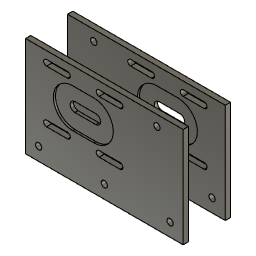
Nema 24 rear mount plate v10 (Autodesk Fusion 360 design; units mm, degrees)
Autodesk Fusion 360 part; units mm, degrees
sketch "Sketch1" plane through (0, 0, 0) normal (0, 1, 0) x (1, 0, 0)
  line L0 (0, 0) -> (150, 0)
  line L1 (150, 0) -> (150, -95)
  line L2 (150, -95) -> (0, -95)
  line L3 (0, -95) -> (0, 0)
  circle A0 centre (125, -85) radius 3
  circle A1 centre (137.5, -12.5) radius 3
  circle A2 centre (75, -12.5) radius 3
  circle A3 centre (12.5, -12.5) radius 3
  circle A4 centre (20, -85) radius 2.75
  line L4 (40, -82.25) -> (20, -82.25)
  line L5 (20.0062, -87.75) -> (40, -87.75)
  circle A5 centre (40, -85) radius 2.75
  circle A6 centre (70, -85) radius 2.75
  line L6 (70, -82.25) -> (90, -82.25)
  line L7 (90, -87.75) -> (70, -87.75)
  circle A7 centre (90, -85) radius 2.75
  circle A8 centre (20, -35) radius 2.75
  line L8 (40, -32.25) -> (20, -32.25)
  line L9 (20, -37.75) -> (40, -37.75)
  circle A9 centre (40, -35) radius 2.75
  circle A10 centre (70, -35) radius 2.75
  line L10 (90, -32.25) -> (70, -32.25)
  line L11 (70, -37.75) -> (90, -37.75)
  circle A11 centre (90, -35) radius 2.75
  line L12 (45, -55.5) -> (65, -55.5)
  line L13 (65, -64.5) -> (45, -64.5)
  circle A12 centre (45, -60) radius 4.5
  circle A13 centre (65, -60) radius 4.5
  circle A14 centre (45, -60) radius 18.5
  line L14 (65.0006, -41.5) -> (45, -41.5)
  circle A15 centre (65, -60) radius 18.5
  line L15 (65.0006, -78.5) -> (45, -78.5)
  dimension "d1" = 150
  dimension "d2" = 95
  dimension "d33" = 6
  dimension "d34" = 6
  dimension "d35" = 6
  dimension "d36" = 6
  dimension "d37" = 5.5
  dimension "d38" = 5.5
  dimension "d39" = 5.5
  dimension "d40" = 5.5
  dimension "d41" = 5.5
  dimension "d42" = 5.5
  dimension "d43" = 5.5
  dimension "d44" = 5.5
  dimension "d45" = 9
  dimension "d46" = 9
  dimension "d49" = 37
  dimension "d50" = 37
  constraint horizontal L0
  constraint vertical L1
  constraint horizontal L2
  constraint vertical L3
  constraint coincident L0.start L3.end
  constraint coincident L5.start A4
  constraint coincident L5.end A5
  constraint tangent L5 A5
  constraint coincident L4.start A5
  constraint coincident L4.end A4
  constraint tangent A4 L4
  constraint horizontal L4
  constraint coincident L7.start A7
  constraint coincident L7.end A6
  constraint tangent A6 L7
  constraint coincident L6.start A6
  constraint coincident L6.end A7
  constraint tangent L6 A7
  constraint parallel L6 L7
  constraint coincident L8.end A8
  constraint tangent A8 L8
  constraint coincident L9.start A8
  constraint coincident L9.end A9
  constraint tangent L9 A9
  constraint parallel L8 L9
  constraint coincident L11.start A10
  constraint coincident L11.end A11
  constraint tangent L11 A11
  constraint coincident L10.start A11
  constraint coincident L10.end A10
  constraint tangent A10 L10
  constraint coincident L12.start A12
  constraint coincident L12.end A13
  constraint tangent L12 A13
  constraint horizontal L12
  constraint coincident L13.start A13
  constraint coincident L13.end A12
  constraint tangent L13 A12
  constraint parallel L12 L13
  constraint coincident L15.start A15
  constraint coincident L15.end A14
  constraint tangent A14 L15
  constraint coincident L14.start A15
  constraint coincident L14.end A14
  constraint tangent A14 L14
  measures "d1" distance of L0.start L0.end
  measures "d2" distance of L0.start L2.end
  measures "d33" diameter of A0
  measures "d34" diameter of A1
  measures "d35" diameter of A2
  measures "d36" diameter of A3
  measures "d37" diameter of A5
  measures "d38" diameter of A4
  measures "d39" diameter of A7
  measures "d40" diameter of A6
  measures "d41" diameter of A9
  measures "d42" diameter of A8
  measures "d43" diameter of A11
  measures "d44" diameter of A10
  measures "d45" diameter of A13
  measures "d46" diameter of A12
  measures "d49" diameter of A15
  measures "d50" diameter of A14
sketch "Sketch2" plane through (0, 0, 0) normal (0, 1, 0) x (1, 0, 0)
  line L0 (0, 0) -> (150, 0)
  line L1 (150, 0) -> (150, -25)
  line L2 (150, -25) -> (0, -25)
  line L3 (0, -25) -> (0, 0)
  circle A0 centre (137.5, -12.5) radius 3
  circle A1 centre (12.5, -12.5) radius 3
  circle A2 centre (75, -12.5) radius 3
  dimension "d3" = 150
  dimension "d4" = 25
  dimension "d19" = 6
  dimension "d20" = 6
  dimension "d21" = 6
  constraint horizontal L0
  constraint vertical L1
  constraint horizontal L2
  constraint vertical L3
  constraint coincident L0.start L3.end
  measures "d3" distance of L0.start L0.end
  measures "d4" distance of L0.start L2.end
  measures "d19" diameter of A0
  measures "d20" diameter of A1
  measures "d21" diameter of A2
sketch "Sketch3" plane through (0, 0, 0) normal (0, 1, 0) x (1, 0, 0)
  line L0 (150, -25) -> (100, -25)
  line L1 (100, -25) -> (100, -75)
  line L2 (100, -75) -> (150, -75)
  line L3 (150, -75) -> (150, -25)
  line L4 (100, -75) -> (150, -75)
  line L5 (150, -75) -> (150, -110)
  line L6 (150, -110) -> (100, -110)
  line L7 (100, -110) -> (100, -75)
  circle A0 centre (125, -85) radius 3
  point P0 (150, -25)
  dimension "d5" = 50
  dimension "d6" = 50
  dimension "d7" = 50
  dimension "d8" = 35
  dimension "d22" = 6
  constraint horizontal L0
  constraint vertical L1
  constraint horizontal L2
  constraint vertical L3
  constraint coincident P0 L0.start
  constraint horizontal L4
  constraint vertical L5
  constraint horizontal L6
  constraint vertical L7
  measures "d5" distance of P0 L0.end
  measures "d6" distance of P0 L2.end
  measures "d7" distance of L1.end L2.end
  measures "d8" distance of L1.end L6.end
  measures "d22" diameter of A0
sketch "Sketch4" plane through (0, 0, 0) normal (0, 1, 0) x (1, 0, 0)
  line L0 (95, -30) -> (15, -30)
  line L1 (15, -30) -> (15, -90)
  line L2 (15, -90) -> (95, -90)
  line L3 (95, -90) -> (95, -30)
  circle A0 centre (65, -60) radius 4.5
  circle A1 centre (65, -60) radius 18.5
  circle A2 centre (40, -85) radius 2.75
  circle A3 centre (90, -85) radius 2.75
  circle A4 centre (40, -35) radius 2.75
  circle A5 centre (90, -35) radius 2.75
  circle A6 centre (20, -35) radius 2.75
  circle A7 centre (20, -85) radius 2.75
  circle A8 centre (70, -85) radius 2.75
  circle A9 centre (70, -35) radius 2.75
  line L4 (20.0062, -87.75) -> (40, -87.75)
  line L5 (40, -82.25) -> (20, -82.25)
  line L6 (90, -87.75) -> (70, -87.75)
  line L7 (70, -82.25) -> (90, -82.25)
  line L8 (70, -37.75) -> (90, -37.75)
  line L9 (90, -32.25) -> (70, -32.25)
  line L10 (40, -32.25) -> (20, -32.25)
  line L11 (20, -37.75) -> (40, -37.75)
  circle A10 centre (45, -60) radius 4.5
  circle A11 centre (45, -60) radius 18.5
  line L12 (65.0006, -78.5) -> (45, -78.5)
  line L13 (65.0006, -41.5) -> (45, -41.5)
  line L14 (45, -55.5) -> (65, -55.5)
  line L15 (65, -64.5) -> (45, -64.5)
  dimension "d9" = 80
  dimension "d10" = 60
  dimension "d11" = 9
  dimension "d12" = 37
  dimension "d13" = 5.5
  dimension "d14" = 5.5
  dimension "d15" = 5.5
  dimension "d16" = 5.5
  dimension "d23" = 5.5
  dimension "d24" = 5.5
  dimension "d25" = 5.5
  dimension "d26" = 5.5
  dimension "d27" = 9
  dimension "d28" = 37
  constraint horizontal L0
  constraint vertical L1
  constraint horizontal L2
  constraint vertical L3
  constraint concentric A0 A1
  constraint coincident A7 L4.start
  constraint coincident A2 L4.end
  constraint tangent A2 L4
  constraint coincident A2 L5.start
  constraint coincident A7 L5.end
  constraint tangent A7 L5
  constraint horizontal L5
  constraint coincident A3 L6.start
  constraint coincident A8 L6.end
  constraint tangent A8 L6
  constraint perpendicular L3 L6
  constraint coincident A8 L7.start
  constraint coincident A3 L7.end
  constraint tangent A3 L7
  constraint parallel L6 L7
  constraint coincident A9 L8.start
  constraint coincident A5 L8.end
  constraint tangent A5 L8
  constraint parallel L2 L8
  constraint coincident A5 L9.start
  constraint coincident A9 L9.end
  constraint tangent A9 L9
  constraint parallel L2 L9
  constraint coincident A6 L10.end
  constraint tangent A6 L10
  constraint parallel L0 L10
  constraint coincident A6 L11.start
  constraint coincident A4 L11.end
  constraint tangent A4 L11
  constraint parallel L10 L11
  constraint coincident A1 L12.start
  constraint coincident A11 L12.end
  constraint tangent A11 L12
  constraint coincident A1 L13.start
  constraint coincident A11 L13.end
  constraint tangent A11 L13
  constraint coincident A10 L14.start
  constraint coincident A0 L14.end
  constraint tangent A0 L14
  constraint horizontal L14
  constraint coincident A0 L15.start
  constraint coincident A10 L15.end
  constraint tangent A10 L15
  constraint parallel L14 L15
  measures "d9" distance of L0.start L0.end
  measures "d10" distance of L0.start L2.end
  measures "d11" diameter of A0
  measures "d12" diameter of A1
  measures "d13" diameter of A2
  measures "d14" diameter of A3
  measures "d15" diameter of A4
  measures "d16" diameter of A5
  measures "d23" diameter of A6
  measures "d24" diameter of A7
  measures "d25" diameter of A8
  measures "d26" diameter of A9
  measures "d27" diameter of A10
  measures "d28" diameter of A11
extrude "Extrude4" add sketch "Sketch1" along normal blind 5 contours L0 L1 L2 L3 | L12 L13 A12 A14 A15 | L12 A14 A15 | L12 L13 A13 A14 A15 | A14 L14 A15 | L13 A14 A15 | A14 A15 L15 makes body 1
extrude "Extrude5" cut sketch "Sketch1" along normal blind 2 contours L12 L13 A12 A14 A15 | L12 A14 A15 | L12 L13 A13 A14 A15 | A14 L14 A15 | L13 A14 A15 | A14 A15 L15 bodies 1
copy_body "CopyPasteBodies1" bodies 1 makes body 2
move_body "Move1" bodies 2 to x (1, 0, 0) y (0, 1, 0) z (0, 0, 1) at (0, 40, 0)
mirror "Mirror1" about plane through (0, 0, 0) normal (1, 0, 0) of bodies 2 makes body 3
move_body "Move2" bodies 3 to x (1, 0, 0) y (0, 1, 0) z (0, 0, 1) at (150, 0, 0)
hidden bodies 2
equation "d9 = 60 mm + 20 mm"
named bodies: "Motor Plate Right", "Motor Plate Left"
